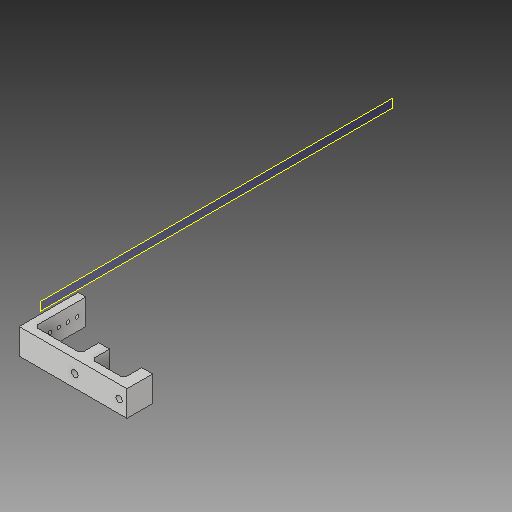
# Autodesk Inventor part: Neje_Endrole_Adapter
Saved by Autodesk Inventor 2019.4 (Build 234330000, 330)
## iProperties
Created: 2021-09-21
Part Number: Neje_Endrole_Adapter
Material: Generic
Document SubType Name: Modeling
Designer: diederichbenedict
Density: 1 g/cm^3
Appearance: Default
Author: diederichbenedict
Autodesk Inventor part; units mm, degrees
ref_plane "YZ Plane" through (0, 0, 0) normal (1, 0, 0) x (0, 1, 0)
ref_plane "XZ Plane" through (0, 0, 0) normal (0, 1, 0) x (-1, 0, 0)
ref_plane "XY Plane" through (0, 0, 0) normal (0, 0, 1) x (1, 0, 0)
ref_plane "Work Plane1" through (-10, 24.3059, -250) normal (-1, 0, 0) x (0, -1, 0)
sketch "Sketch1" plane through (-10, 24.3059, -250) normal (-1, 0, 0) x (0, -1, 0)
  line L0 (28.3059, 0) -> (34.3059, 0) construction
  line L1 (34.3059, 0) -> (34.3059, 250) construction
  line L2 (28.3059, 250) -> (34.3059, 250) construction
  line L3 (28.3059, 0) -> (28.3059, 250) construction
  line L4 (14.3059, 0) -> (20.3059, 0) construction
  line L5 (20.3059, 0) -> (20.3059, 250) construction
  line L6 (14.3059, 250) -> (20.3059, 250) construction
  line L7 (14.3059, 0) -> (14.3059, 250) construction
  line L8 (14.3059, 226.7529) -> (34.3059, 226.7529) construction
  line L9 (34.3059, 226.7529) -> (34.3059, 266.7529) construction
  line L10 (34.3059, 266.7529) -> (14.3059, 266.7529) construction
  line L11 (14.3059, 266.7529) -> (14.3059, 226.7529) construction
  line L12 (14.3059, 266.7529) -> (34.3059, 266.7529) construction
  line L13 (34.3059, 266.7529) -> (34.3059, 226.7529) construction
  line L14 (34.3059, 226.7529) -> (14.3059, 226.7529) construction
  line L15 (14.3059, 226.7529) -> (14.3059, 266.7529) construction
  line L16 (14.3059, 266.7529) -> (34.3059, 266.7529)
  line L17 (34.3059, 266.7529) -> (34.3059, 226.7529)
  line L18 (34.3059, 226.7529) -> (14.3059, 226.7529)
  line L19 (14.3059, 226.7529) -> (14.3059, 266.7529)
  circle A0 centre (24.3059, 261.7529) radius 1.4
  circle A1 centre (24.3059, 254.7529) radius 1.4
  circle A2 centre (24.3059, 247.7529) radius 1.4
  circle A3 centre (24.3059, 240.7529) radius 1.4
  circle A4 centre (24.3059, 233.7529) radius 1.4
  circle A5 centre (24.3059, 226.7529) radius 1.4
  point P0 (24.3059, 250)
  dimension "d0" = 40
  dimension "d1" = 20
  dimension "d2" = 2.8
  dimension "d3" = 5
  dimension "d4" = 10
  dimension "d7" = 7
  constraints: 24 end point, 6 centre point, 6 parallel, 3 horizontal, 3 perpendicular, 1 point on line, 1 vertical, 10 other
  measures "d0" distance of L9.end L8.end
  measures "d1" distance between parallel lines of L11 L9
  measures "d2" diameter of A0
  measures "d3" distance from line of A0.centre L10
  measures "d4" distance from line of L11 A0.centre
  measures "d7" distance of A0.centre A1.centre
extrude "Extrusion1" add sketch "Sketch1" along normal blind 6 contours L16 L17 L18 A5 L19 | A5 L18 picked at (24.759, 226.8646)
sketch "Sketch2" plane through (-10, 10, 16.7529) normal (0, 1, 0) x (1, 0, 0)
  line L0 (0, 0) -> (0, 40) projected
  line L1 (0, 40) -> (-6, 40) projected
  line L2 (-6, 0) -> (-6, 40) projected
  line L3 (0, 0) -> (-6, 0) projected
  line L4 (-6, 40) -> (-6, 0) projected
  line L5 (-6, 0) -> (78, 0)
  line L6 (78, 0) -> (78, -6)
  line L7 (78, -6) -> (-6, -6)
  line L8 (-6, -6) -> (-6, 0)
  line L9 (36, 0) -> (44.5, 0)
  line L10 (44.5, 0) -> (44.5, 14.0376)
  line L11 (44.5, 14.0376) -> (36, 14.0376)
  line L12 (36, 14.0376) -> (36, 0)
  line L13 (78, 0) -> (69.5, 0)
  line L14 (69.5, 0) -> (69.5, 14.0376)
  line L15 (69.5, 14.0376) -> (78, 14.0376)
  line L16 (78, 14.0376) -> (78, 0)
  point P0 (10, 16.7529)
  dimension "d14" = 84
  dimension "d15" = 6
  dimension "d16" = 8.5
  dimension "d17" = 36
  dimension "d18" = 8.5
  constraints: 24 end point, 6 parallel, 3 horizontal, 3 perpendicular, 1 midpoint
  measures "d14" distance of L6.end L7.end
  measures "d15" distance of L5.end L6.end
  measures "d16" distance of L11.end L10.end
  measures "d17" distance between parallel lines of L12 L0
  measures "d18" distance of L14.end L15.end
extrude "Extrusion2" add sketch "Sketch2" against normal up to surface (20 mm away) contours L5 L6 L7 L8 L3 | L12 L11 L10 L5 | L14 L15 L16 L5
chamfer "Chamfer1" distance 2 angle 45 4 edges at (-10, 0, 16.7529) (26, 0, 16.7529) (59.5, 0, 16.7529) (34.5, 0, 16.7529)
sketch "Sketch3" plane through (34.5, 10, 2.7153) normal (0, 0, -1) x (-1, 0, 0)
  circle A0 centre (7.15, -10) radius 2.55 projected
  circle A1 centre (7.15, -10) radius 5.85 projected
  circle A2 centre (-27.35, -10) radius 5.85 projected
  circle A3 centre (-27.35, -10) radius 2.45
  point P0 (34.5, -10)
  dimension "d26" = 4.9
  constraints: 1 centre point, 1 coincident
  measures "d26" diameter of A3
extrude "Extrusion3" cut sketch "Sketch3" against normal through all contours A0 | A3
body "Solid1"
